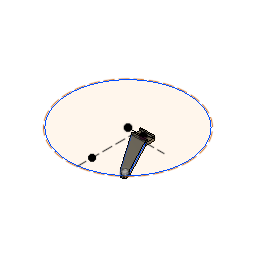
Smart_Useless_Box_lid_arm_v1 (Autodesk Fusion 360 design; units mm, degrees)
Autodesk Fusion 360 part; units mm, degrees
sketch "Sketch1" plane through (0, 0, 0) normal (0, 0, 1) x (1, 0, 0)
  line L0 (5.5, -3.5) -> (-5.5, -3.5)
  line L1 (-5.5, -3.5) -> (-5.5, 3.5)
  line L2 (-5.5, 3.5) -> (5.5, 3.5)
  line L3 (5.5, 3.5) -> (5.5, -3.5)
  line L4 (5.5, -3.5) -> (-5.5, 3.5) construction
  line L5 (-5.5, -3.5) -> (5.5, 3.5) construction
  line L6 (-5.5, 2.75) -> (-5.5, -2.75)
  line L7 (5.5, 2.2) -> (5.5, -2.2)
  line L8 (-5.5, 2.75) -> (5.5, 2.2)
  line L9 (-5.5, -2.75) -> (5.5, -2.2)
  circle A0 centre (0, 0) radius 0.8
  line L10 (-5.5, -3.5) -> (20, -3.5) construction
  line L11 (20, -31.9548) -> (20, -33)
  line L12 (18, -35) -> (17.9246, -35)
  line L13 (-5.5, -46.9761) -> (-5.5, -3.5) construction
  circle A1 centre (-12, 0) radius 47.4236 construction
  line L14 (0, 0) -> (-12, 0)
  line L15 (5.5, -3.5) -> (19.6582, -30.5642)
  line L16 (-5.5, -3.5) -> (15.4597, -33.7101)
  arc A2 (18, -35) -> (20, -33) centre (18, -33) ccw
  circle A3 centre (-12, 0) radius 46.596
  arc A4 (15.4597, -33.7101) -> (17.9246, -35) centre (17.9246, -32) ccw
  arc A5 (20, -31.9548) -> (19.6582, -30.5642) centre (17, -31.9548) ccw
  point P0 (-5.5, -35)
  dimension "d1" = 11
  dimension "d2" = 7
  dimension "d3" = 5.5
  dimension "d4" = 4.4
  dimension "d5" = 1.6
  dimension "d16" = 35
  dimension "d17" = 20
  dimension "d19" = 12
  dimension "d20" = 11.9761
  dimension "d21" = 2
  dimension "d22" = 3
  constraint perpendicular L0 L1
  constraint parallel L0 L2
  constraint parallel L1 L3
  constraint horizontal L0
  constraint coincident L4 A0.centre
  constraint coincident L5 A0.centre
  constraint coincident A0.centre L14.start
  constraint vertical L6
  constraint midpoint L1 L6
  constraint vertical L7
  constraint midpoint L3 L7
  constraint horizontal L10
  constraint vertical L11
  constraint horizontal L12
  constraint vertical L13
  constraint horizontal L14
  constraint coincident A1.centre L14.end
  constraint coincident A1 L13.start
  constraint coincident P0 L13
  constraint tangent L12 A2
  constraint tangent L11 A2
  constraint concentric A1 A3
  constraint coincident P0 L12
  constraint tangent L16 A4
  constraint tangent L12 A4
  constraint coincident L10.end L11
  constraint tangent L15 A5
  constraint tangent L11 A5
  constraint equal A4 A5
  measures "d1" distance of L1.end L2.end
  measures "d2" distance of L0.end L1.end
  measures "d3" distance of L6.start L6.end
  measures "d4" distance of L7.start L7.end
  measures "d5" diameter of A0
  measures "d16" distance of A0.centre L12
  measures "d17" distance of A0.centre L11
  measures "d19" distance of A0.centre A1.centre
  measures "d20" distance of P0 L13.start
  measures "d21" radius of A2
  measures "d22" radius of A4
extrude "Extrude1" add sketch "Sketch1" along normal blind 1.6 contours L0 L1 L3 L9 | L1 L2 L3 L8 makes body 1 at (-1.8333, 2.5667, 0.5333) makes body 2 at (-1.8333, -2.5667, 0.5333)
extrude "Extrude2" add sketch "Sketch1" against normal blind 2.1 contours L0 L1 L3 L9 | L1 L3 L6 L7 L8 L9 | L1 L2 L3 L8 bodies 2 1
extrude "Extrude5" add sketch "Sketch1" along normal up to surface (1.6 mm away) contours L0 L11 L12 L15 L16 A2 A3 A4 A5 bodies 2
extrude "Extrude6" add 1 faces at (5.1532, -13.57, 0) along direction (0, 0, -1) up to surface (2.1 mm away) on bodies 2 bodies 2
